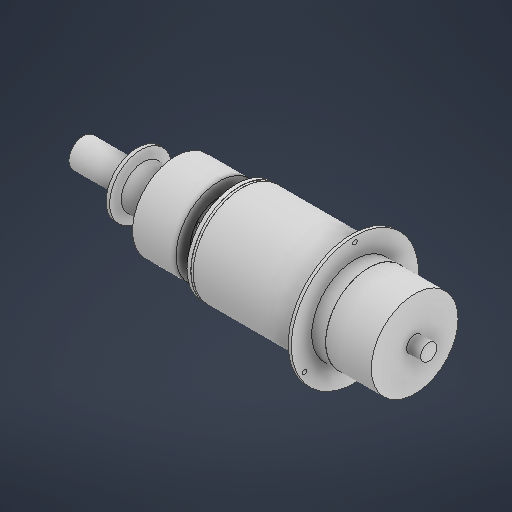
# Autodesk Inventor part: STI Hybrid 98 Cryocooler - Full Flange
Saved by Autodesk Inventor 2026 (Build 300175050, 175E)
## iProperties
Created: 2024-04-30
Part Number: STI Hybrid 98 Cryocooler - Full Flange
Material: Generic
Document SubType Name: Modeling
Designer: incep
Density: 1 g/cm^3
Appearance: Default
Author: incep
Autodesk Inventor part; units mm, degrees
sketch "Sketch1" plane through (0, 0, 0) normal (0, 1, 0) x (-1, 0, 0)
  line L0 (0, 0) -> (-303.89, 0)
  line L1 (0, 0) -> (0, -12.7)
  line L2 (0, -12.7) -> (-87.53, -12.7)
  line L3 (-87.53, -12.7) -> (-87.53, -17.315)
  line L4 (-87.53, -17.315) -> (-50.03, -17.315)
  line L5 (-50.03, -17.315) -> (-50.03, -20.525)
  line L6 (-50.03, -20.525) -> (-47.53, -20.525)
  line L7 (-47.53, -20.525) -> (-47.53, -27.45)
  line L8 (-47.53, -27.45) -> (-50.63, -27.45)
  line L9 (-50.63, -27.45) -> (-52.53, -19.05)
  line L10 (-52.53, -19.05) -> (-81.13, -19.05)
  line L11 (-81.13, -19.05) -> (-81.13, -37.8)
  line L12 (-81.13, -37.8) -> (-119.39, -37.8)
  line L13 (-119.39, -37.8) -> (-119.39, -25.5)
  line L14 (-119.39, -25.5) -> (-134.29, -37.635)
  line L15 (-134.29, -37.635) -> (-134.29, -43.07)
  line L16 (-134.29, -43.07) -> (-137.79, -43.07)
  line L17 (-137.79, -43.07) -> (-137.79, -43.28)
  line L18 (-137.79, -43.28) -> (-139.89, -43.28)
  line L19 (-139.89, -43.28) -> (-139.89, -43.175)
  line L20 (-139.89, -43.175) -> (-236.29, -43.175)
  line L21 (-236.29, -43.175) -> (-236.29, -56)
  line L22 (-236.29, -56) -> (-238.99, -56)
  line L23 (-238.99, -56) -> (-238.99, 0)
  line L24 (-251.3, 0) -> (-251.3, -38.15)
  line L25 (-251.3, -38.15) -> (-291.54, -38.15)
  line L26 (-291.54, -38.15) -> (-291.54, -7.165)
  line L27 (-291.54, -7.165) -> (-303.89, -7.165)
  line L28 (-303.89, -7.165) -> (-303.89, 0)
  line L29 (-238.99, -38) -> (-251.3, -38)
  line L30 (-251.3, -38) -> (-251.3, 0)
  line L31 (-251.3, 0) -> (-238.99, 0)
  line L32 (-238.99, 0) -> (-238.99, -38)
  dimension "d0" = 303.89
  dimension "d1" = 12.7
  dimension "d2" = 87.53
  dimension "d3" = 4.615
  dimension "d4" = 37.5
  dimension "d5" = 3.21
  dimension "d6" = 2.5
  dimension "d7" = 27.45
  dimension "d8" = 3.1
  dimension "d9" = 5
  dimension "d10" = 19.05
  dimension "d11" = 30.5
  dimension "d12" = 37.8
  dimension "d13" = 38.26
  dimension "d14" = 12.3
  dimension "d16" = 14.9
  dimension "d17" = 37.635
  dimension "d18" = 43.07
  dimension "d19" = 3.5
  dimension "d20" = 43.28
  dimension "d21" = 2.1
  dimension "d22" = 43.175
  dimension "d24" = 56
  dimension "d25" = 104.7
  dimension "d26" = 12.31
  dimension "d27" = 157.25
  dimension "d28" = 38.15
  dimension "d29" = 90
  dimension "d30" = 7.165
  dimension "d31" = 12.35
  dimension "d54" = 2.7
  dimension "d55" = 38
  dimension "d77" = 25.5
  dimension "d78" = 102
  constraints: 66 end point, 13 perpendicular, 9 vertical, 4 horizontal, 4 parallel, 3 point on line
  measures "d0" distance of L0.start L0.end
  measures "d1" distance of L0.start L1.end
  measures "d2" distance of L1.end L2.end
  measures "d3" distance of L2.end L3.end
  measures "d4" distance of L3.end L4.end
  measures "d5" distance of L4.end L5.end
  measures "d6" distance of L5.end L6.end
  measures "d7" vertical distance of L0.start L7.end
  measures "d8" distance of L7.end L8.end
  measures "d9" distance from line of L9.end L7
  measures "d10" distance from line of L10 L0.start
  measures "d11" distance from line of L11 L8.end
  measures "d12" distance from line of L0.start L12
  measures "d13" distance of L11.end L12.end
  measures "d14" distance of L12.end L13.end
  measures "d16" distance between parallel lines of L15 L13
  measures "d17" distance from line of L14.end L0
  measures "d18" distance between parallel lines of L0 L16
  measures "d19" distance of L15.end L16.end
  measures "d20" distance between parallel lines of L0 L18
  measures "d21" distance of L17.end L18.end
  measures "d22" distance between parallel lines of L0 L20
  measures "d24" distance between parallel lines of L0 L22
  measures "d25" distance between parallel lines of L23 L15
  measures "d26" distance between parallel lines of L24 L23
  measures "d27" distance from line of L25.end L15
  measures "d28" distance between parallel lines of L0 L25
  measures "d29" angle of L27 L26
  measures "d30" distance of L27.end L0.end
  measures "d31" distance of L26.end L27.end
  measures "d54" distance of L22.end L21.end
  measures "d55" distance between parallel lines of L0 L29
  measures "d77" distance from line of L0 L13.end
  measures "d78" distance from line of L21 L15.end
revolve "Revolution1" add sketch "Sketch1" angle 360 about axis through (0, 0, 0) along (1, 0, 0)
ref_plane "Work Plane1" through (236.99, 0, 0) normal (1, 0, 0) x (0, 0, -1)
ref_plane "Work Plane2" through (236.99, 52.5583, -19.3295) normal (0, 0.9385405, -0.3451692) x (-1, 0, 0)
sketch "Sketch6" plane through (238.99, 0, 0) normal (1, 0, 0) x (0, 0, -1)
  line L0 (44.25, -25.5477) -> (-44.25, -25.5477)
  line L1 (-44.25, -25.5477) -> (0, 51.0955)
  line L2 (0, 51.0955) -> (44.25, -25.5477)
  circle A0 centre (0, 51.0955) radius 2
  circle A1 centre (44.25, -25.5477) radius 2
  circle A2 centre (-44.25, -25.5477) radius 2
  point P0 (0, 0)
  point P1 (0, 0)
  dimension "d56" = 4
  dimension "d57" = 88.5
  constraints: 6 end point, 4 coincident, 3 centre point, 2 equal radius, 1 horizontal, 7 other
  measures "d56" diameter of A0
  measures "d57" distance of L0.start L0.end
extrude "Extrusion3" cut sketch "Sketch6" against normal up to surface (2.7 mm away) contours A2 L1 L0 | L0 L1 A2 | A1 L2 L0 | L0 L2 A1 | A0 L2 L1 | L1 L2 A0
ref_plane "Work Plane3" through (128.29, 0, 0) normal (-1, 0, 0) x (0, 0, 1)
sketch "Sketch7" plane through (128.29, 0, 0) normal (-1, 0, 0) x (0, 0, 1)
  circle A0 centre (0, 51.0955) radius 2 projected
  circle A1 centre (0, 0) radius 25.5 projected
  circle A2 centre (0, 0) radius 37.635 projected
  circle A3 centre (0, 0) radius 32.635 construction
  circle A4 centre (0, 32.635) radius 2
  circle A5 centre (25.2927, 20.6234) radius 2
  dimension "d61" = 5
  dimension "d62" = 4
  dimension "d64" = 28
  constraints: 3 centre point, 2 point on circle, 1 equal radius, 1 vertical alignment
  measures "d61" radial gap between concentric circles of A2 A3
  measures "d62" diameter of A4
  measures "d64" distance of A4.centre A5.centre
extrude "Extrusion4" add sketch "Sketch7" along normal mid plane 3 contours A4 | A5
ref_plane "Work Plane4" through (226.29, 0, 0) normal (-1, 0, 0) x (0, 0, 1)
sketch "Sketch8" plane through (226.29, 0, 0) normal (-1, 0, 0) x (0, 0, 1)
  circle A0 centre (0, 0) radius 43.175 projected
  circle A1 centre (0, 0) radius 43.175 projected
  circle A2 centre (-44.25, -25.5477) radius 2 projected
  line L0 (-44.25, -25.5477) -> (-37.3906, -21.5875) construction
  point P0 (-23.6509, -36.1209)
  dimension "d68" = 20
  constraints: 2 end point, 2 point on circle, 1 line through centre
  measures "d68" distance of A1.start L0.end
ref_plane "Work Plane5" through (226.29, -36.1209, -23.6509) normal (0, -0.8366152, -0.547791) x (1, 0, 0)
sketch "Sketch9" plane through (226.29, -36.1209, -23.6509) normal (0, -0.8366152, -0.547791) x (1, 0, 0)
  circle A0 centre (0, 0) radius 3.1
  point P0 (-226.29, 0)
  dimension "d69" = 6.2
  constraints: 1 centre point
  measures "d69" diameter of A0
extrude "Extrusion5" add sketch "Sketch9" along normal blind 26 and the other way blind 1
sketch "Sketch10" plane through (226.29, -57.8729, -37.8934) normal (0, -0.8366152, -0.547791) x (1, 0, 0)
  circle A0 centre (0, 0) radius 3.1 projected
  circle A1 centre (0, 0) radius 7
  point P0 (-226.29, 0)
  dimension "d74" = 14
  constraints: 1 centre point, 1 coincident
  measures "d74" diameter of A1
extrude "Extrusion6" add sketch "Sketch10" against normal blind 13 contours A0 | A1
body "Solid1"
